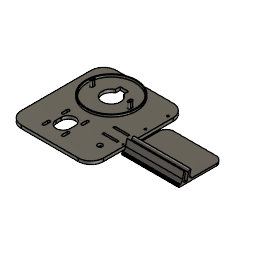
Nasty_Mounting (Autodesk Fusion 360 design; units mm, degrees)
Autodesk Fusion 360 part; units mm, degrees
sketch "bovenkant" plane through (0, 0, 0) normal (0, 0, 1) x (1, 0, 0)
  circle A0 centre (-96.358, 36.4115) radius 1.25
  circle A1 centre (-48.858, 36.4115) radius 1.25
  circle A2 centre (-96.358, -11.0885) radius 1.25
  circle A3 centre (-48.858, -11.0885) radius 1.25
  circle A4 centre (-72.6345, 12.688) radius 14.5
  line L0 (-66.1493, 33.1295) -> (-79.0952, 33.1295)
  line L1 (-79.0952, 33.1295) -> (-79.0952, 25.6691)
  line L2 (-66.1493, 25.6569) -> (-66.1493, 33.1295)
  line L3 (-72.6345, 12.688) -> (-74.3845, 12.688)
  line L4 (-72.6345, 12.688) -> (-70.8845, 12.688)
  line L5 (-104.9345, 14.288) -> (-104.9345, 11.088)
  arc A5 (-104.9345, 11.088) -> (-100.1345, 11.088) centre (-102.5345, 11.088) ccw
  line L6 (-100.1345, 11.088) -> (-100.1345, 14.288)
  arc A6 (-100.1345, 14.288) -> (-104.9345, 14.288) centre (-102.5345, 14.288) ccw
  arc A7 (-104.6845, 11.088) -> (-100.3845, 11.088) centre (-102.5345, 11.088) ccw
  line L7 (-100.3845, 11.088) -> (-100.3845, 14.2881)
  arc A8 (-100.3845, 14.2881) -> (-104.6845, 14.288) centre (-102.5345, 14.288) ccw
  line L8 (-104.6845, 14.288) -> (-104.6845, 11.088)
  arc A9 (-71.0345, -19.612) -> (-71.0345, -14.812) centre (-71.0345, -17.212) ccw
  line L9 (-71.0345, -14.812) -> (-74.2345, -14.812)
  arc A10 (-74.2345, -15.062) -> (-74.2345, -19.362) centre (-74.2345, -17.212) ccw
  arc A11 (-71.0345, -19.362) -> (-71.0345, -15.062) centre (-71.0345, -17.212) ccw
  line L10 (-74.2345, -19.362) -> (-71.0345, -19.362)
  line L11 (-74.2345, -19.612) -> (-71.0345, -19.612)
  arc A12 (-74.2345, -14.812) -> (-74.2345, -19.612) centre (-74.2345, -17.212) ccw
  line L12 (-71.0345, -15.062) -> (-74.2345, -15.062)
  arc A13 (-40.3345, 14.288) -> (-45.1345, 14.288) centre (-42.7345, 14.288) ccw
  line L13 (-45.1345, 14.288) -> (-45.1345, 11.088)
  arc A14 (-44.8845, 11.088) -> (-40.5845, 11.088) centre (-42.7345, 11.088) ccw
  arc A15 (-40.5845, 14.2881) -> (-44.8845, 14.288) centre (-42.7345, 14.288) ccw
  line L14 (-40.5845, 11.088) -> (-40.5845, 14.2881)
  line L15 (-40.3345, 11.088) -> (-40.3345, 14.288)
  arc A16 (-45.1345, 11.088) -> (-40.3345, 11.088) centre (-42.7345, 11.088) ccw
  line L16 (-44.8845, 14.288) -> (-44.8845, 11.088)
  arc A17 (-74.2345, 44.988) -> (-74.2345, 40.188) centre (-74.2345, 42.588) ccw
  line L17 (-74.2345, 40.188) -> (-71.0345, 40.188)
  arc A18 (-71.0345, 40.438) -> (-71.0345, 44.738) centre (-71.0345, 42.588) ccw
  arc A19 (-74.2345, 44.738) -> (-74.2345, 40.438) centre (-74.2345, 42.588) ccw
  line L18 (-71.0345, 44.738) -> (-74.2345, 44.738)
  line L19 (-71.0345, 44.988) -> (-74.2345, 44.988)
  arc A20 (-71.0345, 40.188) -> (-71.0345, 44.988) centre (-71.0345, 42.588) ccw
  line L20 (-74.2345, 40.438) -> (-71.0345, 40.438)
  circle A21 centre (-72.6345, 12.688) radius 37.5
  circle A22 centre (-72.6345, 12.688) radius 39.75
  circle A23 centre (-102.5345, 12.688) radius 1.6
  circle A24 centre (-42.7345, 12.688) radius 1.6
  point P0 (-72.6345, 12.688)
  point P1 (-72.6345, 12.688)
  dimension "d4" = 2.5
  dimension "d7" = 47.5
  dimension "d8" = -47.5
  dimension "d9" = 29
  dimension "d12" = 7.4725
  dimension "d19" = -0.25
  dimension "d21" = 360
  dimension "d22" = 27.5
  dimension "d23" = 75
  dimension "d24" = 79.5
  dimension "d41" = 360
  dimension "d44" = 3.2
  constraint horizontal L0
  constraint perpendicular L0 L1
  constraint parallel L1 L2
  constraint coincident P1 P0
  constraint coincident A4 L1.end
  constraint coincident A4 L2.start
  constraint horizontal L3
  constraint coincident P0 A4.centre
  constraint horizontal L4
  constraint tangent L5 A5
  constraint tangent A5 L6
  constraint parallel L5 L6
  constraint tangent L6 A6
  constraint tangent L5 A6
  constraint coincident A5.centre A23
  constraint coincident A6.centre A23
  measures "d4" diameter of A0
  measures "d9" diameter of A4
  measures "d12" distance of L0.start L2.start
  measures "d22" distance of P1 L6
  measures "d23" diameter of A21
  measures "d24" diameter of A22
  measures "d44" diameter of A23
extrude "Extrude1" add sketch "bovenkant" against normal blind 3 contours A0 | A1 | A2 | A3 | A4 | A4 L0 L1 L2 | L5 A5 L6 A6 | A7 L7 A8 L8 | A9 L9 L11 A12 | A10 A11 L10 L12 | A13 L13 L15 A16 | A14 A15 L14 L16 | A17 L17 L19 A20 | A18 A19 L18 L20 | A21 | A22 | A23 | A24 makes body 1
extrude "Extrude3" add sketch "bovenkant" along normal blind 9 separate body contours A7 L7 A8 L8 | A14 A15 L14 L16 | A23 | A24 makes body 2 at (-42.1522, 9.0184, 3) makes body 3 at (-102.1611, 16.4054, 6)
ref_plane "WorkPlane1" through (-96.358, 36.4115, 3) normal (0, 0, 1) x (1, 0, 0)
sketch "rand" plane through (0, 0, 3) normal (0, 0, 1) x (1, 0, 0)
  circle A0 centre (-72.6345, 12.688) radius 39.75
  circle A1 centre (-72.6345, 12.688) radius 38.25
  dimension "d32" = -1.5
extrude "Extrude4" add sketch "rand" against normal up to surface (3 mm away) bodies 1
chamfer "Chamfer1" distance 0.5 distance2 3 1 edges at (-108.296, -1.1438, 0) measured on face at (-75.4716, 23.995, 0) on bodies 1
extrude "Extrude5" cut sketch "bovenkant" against normal up to surface (3 mm away) contours A4 | A4 L0 L1 L2 bodies 1
combine "Combine1" operation add target body 3 tool bodies 1 2
extrude "Extrude6" cut sketch "bovenkant" along normal blind 14 and the other way blind 2 contours A23 | A24 bodies 3
sketch "Onderkant" plane through (0, 0, -3) normal (0, 0, -1) x (1, 0, 0)
  arc A0 (-66.1493, -25.6569) -> (-79.0952, -25.6691) centre (-72.6345, -12.688) ccw
  line L0 (-66.1493, -25.6569) -> (-66.1493, -33.1295)
  line L1 (-66.1493, -33.1295) -> (-79.0952, -33.1295)
  line L2 (-79.0952, -33.1295) -> (-79.0952, -25.6691)
  circle A1 centre (-72.6345, -12.688) radius 39.75
  circle A2 centre (-42.7345, -12.688) radius 1.6
  circle A3 centre (-102.5345, -12.688) radius 1.6
  line L3 (-45.6345, -14.3624) -> (-42.7345, -16.0367)
  line L4 (-42.7345, -16.0367) -> (-39.8345, -14.3624)
  line L5 (-39.8345, -14.3624) -> (-39.8345, -11.0137)
  line L6 (-39.8345, -11.0137) -> (-42.7345, -9.3394)
  line L7 (-42.7345, -9.3394) -> (-45.6345, -11.0137)
  line L8 (-45.6345, -11.0137) -> (-45.6345, -14.3624)
  line L9 (-105.4345, -14.3624) -> (-102.5345, -16.0367)
  line L10 (-102.5345, -16.0367) -> (-99.6345, -14.3624)
  line L11 (-99.6345, -14.3624) -> (-99.6345, -11.0137)
  line L12 (-99.6345, -11.0137) -> (-102.5345, -9.3394)
  line L13 (-102.5345, -9.3394) -> (-105.4345, -11.0137)
  line L14 (-105.4345, -11.0137) -> (-105.4345, -14.3624)
  point P0 (-102.5345, -12.688)
  point P1 (-42.7345, -12.688)
  point P2 (-42.7345, -12.688)
  point P3 (-102.5345, -12.688)
  dimension "d45" = 2.9
  dimension "d46" = 2.9
  constraint coincident P2 P1
  constraint coincident P3 P0
  measures "d45" distance of P2 L8
  measures "d46" distance of P3 L14
sketch "maten_hardware" plane through (0, 0, 0) normal (0, 0, 1) x (1, 0, 0)
  circle A0 centre (-72.6345, 12.688) radius 39.75
  circle A1 centre (-72.6345, 12.688) radius 39.75
  line L0 (-83.9345, -55.312) -> (-83.9345, -63.312)
  arc A2 (-83.9345, -63.312) -> (-61.4345, -63.312) centre (-72.6845, -63.312) ccw
  line L1 (-61.4345, -63.312) -> (-61.4345, -55.312)
  arc A3 (-61.4345, -55.312) -> (-83.9345, -55.312) centre (-72.6845, -55.312) ccw
  line L2 (-72.6845, -55.312) -> (-72.6845, -63.312) construction
  line L3 (-57.4289, -44.062) -> (-57.4289, -40.062)
  line L4 (-57.4289, -44.062) -> (-57.4289, -48.062)
  line L5 (-59.3289, -40.062) -> (-59.3289, -48.062)
  arc A4 (-59.3289, -48.062) -> (-55.5289, -48.062) centre (-57.4289, -48.062) ccw
  line L6 (-55.5289, -48.062) -> (-55.5289, -40.062)
  arc A5 (-55.5289, -40.062) -> (-59.3289, -40.062) centre (-57.4289, -40.062) ccw
  line L7 (-57.4289, -40.062) -> (-57.4289, -48.062) construction
  line L8 (-50.6309, -20.4164) -> (-50.6309, -84.1336)
  line L9 (-50.6309, -84.1336) -> (-94.6381, -84.1336)
  line L10 (-94.6381, -84.1336) -> (-94.6381, -20.4164)
  line L11 (-87.9289, -44.062) -> (-87.9289, -48.062)
  line L12 (-87.9289, -40.062) -> (-87.9289, -48.062) construction
  line L13 (-87.9289, -44.062) -> (-87.9289, -40.062)
  line L14 (-86.0289, -48.062) -> (-86.0289, -40.062)
  arc A6 (-86.0289, -40.062) -> (-89.8289, -40.062) centre (-87.9289, -40.062) ccw
  line L15 (-89.8289, -40.062) -> (-89.8289, -48.062)
  arc A7 (-89.8289, -48.062) -> (-86.0289, -48.062) centre (-87.9289, -48.062) ccw
  line L16 (-57.4289, -74.562) -> (-57.4289, -78.562)
  line L17 (-57.4289, -70.562) -> (-57.4289, -78.562) construction
  line L18 (-57.4289, -74.562) -> (-57.4289, -70.562)
  line L19 (-55.5289, -78.562) -> (-55.5289, -70.562)
  arc A8 (-55.5289, -70.562) -> (-59.3289, -70.562) centre (-57.4289, -70.562) ccw
  line L20 (-59.3289, -70.562) -> (-59.3289, -78.562)
  arc A9 (-59.3289, -78.562) -> (-55.5289, -78.562) centre (-57.4289, -78.562) ccw
  line L21 (-87.9289, -74.562) -> (-87.9289, -78.562)
  line L22 (-87.9289, -70.562) -> (-87.9289, -78.562) construction
  line L23 (-87.9289, -74.562) -> (-87.9289, -70.562)
  line L24 (-86.0289, -78.562) -> (-86.0289, -70.562)
  arc A10 (-86.0289, -70.562) -> (-89.8289, -70.562) centre (-87.9289, -70.562) ccw
  line L25 (-89.8289, -70.562) -> (-89.8289, -78.562)
  arc A11 (-89.8289, -78.562) -> (-86.0289, -78.562) centre (-87.9289, -78.562) ccw
  line L26 (4.0655, -25.2683) -> (-32.3045, -25.2683)
  line L27 (-32.3045, -25.2683) -> (-32.3045, -45.5883)
  line L28 (-32.3045, -45.5883) -> (4.0655, -45.5883)
  line L29 (4.0655, -45.5883) -> (4.0655, -25.2683)
  line L30 (2.0955, -27.2683) -> (2.0955, -43.5883)
  line L31 (-29.9045, -28.7883) -> (-29.9045, -42.0683)
  circle A12 centre (2.0955, -27.2683) radius 1.15
  circle A13 centre (-29.9045, -28.7883) radius 1.15
  circle A14 centre (-29.9045, -42.0683) radius 1.15
  circle A15 centre (2.0955, -43.5883) radius 1.15
  circle A16 centre (-1.1507, 30.6175) radius 1.6
  circle A17 centre (-36.6507, 30.6175) radius 1.6
  circle A18 centre (-1.1507, -4.8825) radius 1.6
  circle A19 centre (-36.6507, -4.8825) radius 1.6
  line L32 (2.5993, 34.3675) -> (-40.4007, 34.3675)
  line L33 (-40.4007, 34.3675) -> (-40.4007, -8.6325)
  line L34 (-40.4007, -8.6325) -> (2.5993, -8.6325)
  line L35 (2.5993, -8.6325) -> (2.5993, 34.3675)
  line L36 (-8.6345, -56.7369) -> (-21.1345, -56.7369)
  line L37 (-21.1345, -56.7369) -> (-21.1345, -69.2369)
  line L38 (-21.1345, -69.2369) -> (-8.6345, -69.2369)
  line L39 (-8.6345, -69.2369) -> (-8.6345, -56.7369)
  line L40 (-8.6345, -56.7369) -> (-21.1345, -69.2369) construction
  line L41 (-21.1345, -56.7369) -> (-8.6345, -69.2369) construction
  circle A20 centre (-14.8845, -62.9869) radius 3.75
  line L42 (-96.0345, 6.5117) -> (-123.6345, 6.5117)
  line L43 (-123.6345, 6.5117) -> (-123.6345, -57.4883)
  line L44 (-123.6345, -57.4883) -> (-96.0345, -57.4883)
  line L45 (-96.0345, -57.4883) -> (-96.0345, 6.5117)
  line L46 (-29.1045, -25.3683) -> (-5.6045, -25.3683)
  line L47 (-5.6045, -25.3683) -> (-5.6045, -28.3683)
  line L48 (-5.6045, -28.3683) -> (-29.1045, -28.3683)
  line L49 (-29.1045, -28.3683) -> (-29.1045, -25.3683)
  line L50 (-31.2285, -35.4283) -> (-20.6732, -35.4283)
  line L51 (-5.6045, -42.4883) -> (-29.1045, -42.4883)
  line L52 (-29.1045, -42.4883) -> (-29.1045, -45.4883)
  line L53 (-29.1045, -45.4883) -> (-5.6045, -45.4883)
  line L54 (-5.6045, -45.4883) -> (-5.6045, -42.4883)
  line L55 (5.3655, -77.4883) -> (5.3655, 32.5117)
  line L56 (-14.6345, 52.5117) -> (-104.6345, 52.5117)
  line L57 (-124.6345, 32.5117) -> (-124.6345, -77.4883)
  line L58 (-104.6345, -97.4883) -> (-14.6345, -97.4883)
  arc A21 (-104.6345, 52.5117) -> (-124.6345, 32.5117) centre (-104.6345, 32.5117) ccw
  arc A22 (5.3655, 32.5117) -> (-14.6345, 52.5117) centre (-14.6345, 32.5117) ccw
  arc A23 (-124.6345, -77.4883) -> (-104.6345, -97.4883) centre (-104.6345, -77.4883) ccw
  arc A24 (-14.6345, -97.4883) -> (5.3655, -77.4883) centre (-14.6345, -77.4883) ccw
  point P0 (-72.6845, -59.312)
  point P1 (-14.8845, -62.9869)
  point P2 (5.3655, -97.4883)
  point P3 (-124.6345, -97.4883)
  dimension "d53" = 22.5
  dimension "d57" = 4
  dimension "d58" = 4
  dimension "d63" = 3.8
  dimension "d80" = -30.5
  dimension "d81" = -30.5
  dimension "d82" = 36.37
  dimension "d83" = 20.32
  dimension "d88" = 16.32
  dimension "d89" = 2
  dimension "d90" = 1.97
  dimension "d91" = 13.28
  dimension "d92" = 3.52
  dimension "d93" = 2.4
  dimension "d94" = 2.3
  dimension "d95" = 2.3
  dimension "d97" = 2.3
  dimension "d98" = 2.3
  dimension "d102" = 3.2
  dimension "d105" = -35.5
  dimension "d106" = -35.5
  dimension "d107" = 43
  dimension "d108" = 43
  dimension "d109" = 3.75
  dimension "d110" = 3.75
  dimension "d111" = 12.5
  dimension "d112" = 12.5
  dimension "d113" = 7.5
  dimension "d114" = 27.6
  dimension "d115" = 64
  dimension "d118" = 23.5
  dimension "d119" = 3
  dimension "d120" = 0.1
  dimension "d121" = 3.2
  dimension "d122" = 10.16
  dimension "d123" = 130
  dimension "d124" = 20
  dimension "d139" = 150
  dimension "d140" = 1.3
  dimension "d147" = 2.7662
  dimension "d148" = 1
  dimension "d149" = 44.0072
  dimension "d150" = 52
  dimension "d151" = 14
  dimension "d152" = 52
  dimension "d153" = 40
  constraint tangent L0 A2
  constraint tangent A2 L1
  constraint parallel L0 L1
  constraint tangent L1 A3
  constraint tangent L0 A3
  constraint midpoint L2 P0
  constraint tangent L5 A4
  constraint tangent A4 L6
  constraint parallel L5 L6
  constraint tangent L6 A5
  constraint tangent L5 A5
  constraint coincident L4.end A4.centre
  constraint parallel L4 L7
  constraint coincident L3.end A5.centre
  constraint perpendicular L8 L9
  constraint parallel L8 L10
  constraint coincident A1 L8.start
  constraint horizontal L26
  constraint vertical L27
  constraint horizontal L28
  constraint vertical L29
  constraint perpendicular L26 L30
  constraint perpendicular L26 L31
  constraint coincident L30.start A12.centre
  constraint coincident L31.start A13.centre
  constraint coincident L31.end A14.centre
  constraint coincident L30.end A15.centre
  constraint horizontal L32
  constraint vertical L33
  constraint horizontal L34
  constraint vertical L35
  constraint horizontal L36
  constraint perpendicular L36 L37
  constraint parallel L36 L38
  constraint parallel L37 L39
  constraint coincident L40 P1
  constraint coincident L41 P1
  constraint coincident P1 A20.centre
  constraint horizontal L42
  constraint vertical L43
  constraint horizontal L44
  constraint vertical L45
  constraint horizontal L46
  constraint vertical L47
  constraint horizontal L48
  constraint vertical L49
  constraint horizontal L50
  constraint symmetric L46.start L50 L52.end
  constraint symmetric L46.end L50 L53.end
  constraint symmetric L47.end L50 L51.start
  constraint symmetric L48.end L50 L51.end
  constraint perpendicular L55 L56
  constraint parallel L55 L57
  constraint parallel L56 L58
  constraint perpendicular L32 L55
  constraint tangent L56 A21
  constraint tangent L57 A21
  constraint tangent L55 A22
  constraint tangent L56 A22
  constraint equal A21 A22
  constraint coincident P3 L57
  constraint coincident P3 L58
  constraint tangent L57 A23
  constraint tangent L58 A23
  constraint equal A21 A23
  constraint coincident P2 L55
  constraint coincident P2 L58
  constraint tangent L55 A24
  constraint tangent L58 A24
  constraint equal A21 A24
  constraint coincident A0 L10.end
  measures "d53" diameter of A2
  measures "d57" distance of L3.start L3.end
  measures "d58" distance of L3.start L4.end
  measures "d63" diameter of A4
  measures "d82" distance of L26.start L26.end
  measures "d83" distance of L26.start L28.end
  measures "d88" distance of L30.start L30.end
  measures "d89" distance of L26 L30.start
  measures "d90" distance of L29 L30
  measures "d91" distance of L31.start L31.end
  measures "d92" distance of L26 L31.start
  measures "d93" distance of L27 L31
  measures "d94" diameter of A12
  measures "d95" diameter of A13
  measures "d97" diameter of A14
  measures "d98" diameter of A15
  measures "d102" diameter of A16
  measures "d107" distance of L32.start L32.end
  measures "d108" distance of L32.start L34.end
  measures "d109" distance of A16.centre L35
  measures "d110" distance of A16.centre L32
  measures "d111" distance of L37.end L38.end
  measures "d112" distance of L36.end L37.end
  measures "d113" diameter of A20
  measures "d114" distance of L42.start L42.end
  measures "d115" distance of L42.start L44.end
  measures "d118" distance of L46.start L46.end
  measures "d119" distance of L46.start L48.end
  measures "d120" distance of L26 L46
  measures "d121" distance of L27 L49
  measures "d122" distance of L26 L50
  measures "d123" distance of P2 P3
  measures "d124" radius of A21
  measures "d139" distance of L56 L58
  measures "d140" distance of L29 L55
  measures "d147" distance of L35 L55
  measures "d148" distance of L43 L57
  measures "d149" distance of L8 L10
  measures "d150" distance of A0.centre L57
  measures "d151" distance of L39 L55
  measures "d152" distance of L53 L58
  measures "d153" distance of L44 L58
extrude "Extrude8" add sketch "maten_hardware" against normal blind 5 contours A0 A1 L8 L9 L10 | A0 A1 L42 L43 L44 L45 | A0 A1 A17 A19 L32 L34 L35 | A0 A1 A19 | A0 A1 A17 | L26 L27 L28 L29 | A13 L48 L49 | A14 L51 L52 | L36 L37 L38 L39 | L55 L56 L57 L58 A21 A22 A23 A24 picked at (-36.348, -5.0254) picked at (-36.4402, 30.7083) picked at (-30.3145, -29.0044) picked at (-30.3145, -41.8522) bodies 3
extrude "Extrude12" add 1 faces at (-71.6362, 39.5286, -3) along direction (0, 0, -1) up to surface (2 mm away) on bodies 3 bodies 3
ref_plane "WorkPlane2" through (-59.6345, -22.4883, -5) normal (0, 0, -1) x (-1, 0, 0)
sketch "Sketch6" plane through (0, 0, -5) normal (0, 0, -1) x (-1, 0, 0)
  line L0 (123.6345, -57.4883) -> (96.0345, -57.4883)
  line L1 (123.6345, 6.5117) -> (123.6345, -57.4883)
  line L2 (96.0345, -57.4883) -> (96.0345, 6.5117)
  line L3 (96.0345, 6.5117) -> (123.6345, 6.5117)
  line L4 (8.6345, -56.7369) -> (21.1345, -56.7369)
  line L5 (21.1345, -56.7369) -> (21.1345, -69.2369)
  line L6 (21.1345, -69.2369) -> (8.6345, -69.2369)
  line L7 (8.6345, -69.2369) -> (8.6345, -56.7369)
  line L8 (40.4007, -8.6325) -> (-2.5993, -8.6325)
  line L9 (40.4007, 34.3675) -> (40.4007, -8.6325)
  line L10 (-2.5993, 34.3675) -> (40.4007, 34.3675)
  line L11 (-2.5993, -8.6325) -> (-2.5993, 34.3675)
extrude "Extrude10" cut sketch "Sketch6" against normal blind 3.5 bodies 3
sketch "Sketch7" plane through (0, 0, 0) normal (1, 0, 0) x (0, 1, 0)
  line L0 (-91.4917, 4.5771) -> (-93.4917, 4.5771)
  line L1 (-93.9917, 4.0771) -> (-93.9917, -66.1853)
  line L2 (-93.9917, -66.1853) -> (-90.9917, -66.1853)
  line L3 (-90.9917, 2.1282) -> (-90.9917, 4.0771)
  arc A0 (-90.9917, 2.1282) -> (-90.5352, 1.6301) centre (-90.4917, 2.1282) ccw
  arc A1 (-90.9917, 4.0771) -> (-91.4917, 4.5771) centre (-91.4917, 4.0771) ccw
  arc A2 (-93.4917, 4.5771) -> (-93.9917, 4.0771) centre (-93.4917, 4.0771) ccw
  line L4 (-90.9917, -0.4229) -> (-75.3696, -3.8798)
  line L5 (-77.8019, -14.8716) -> (-93.4104, -11.4098)
  line L6 (-93.4104, -11.4098) -> (-90.9917, -0.4229)
  line L7 (-77.152, -11.9349) -> (-91.7977, -8.6941)
  line L8 (-91.7977, -8.6941) -> (-90.6634, -3.5681)
  line L9 (-90.6634, -3.5681) -> (-76.0177, -6.8089)
  line L10 (-75.3696, -3.8798) -> (-76.0177, -6.8089)
  line L11 (-77.152, -11.9349) -> (-77.8019, -14.8716)
  line L12 (-90.8603, 1.7904) -> (-90.9917, -66.1853)
  point P0 (-90.9917, 4.5771)
  point P1 (-93.9917, 4.5771)
  dimension "d131" = 3
  dimension "d134" = 0.5
  dimension "d160" = 16
  dimension "d161" = 11.25
  dimension "d162" = 15
  dimension "d163" = 5.25
  dimension "d164" = 3
  dimension "d165" = 3
  dimension "d166" = 5
  constraint horizontal L0
  constraint vertical L1
  constraint horizontal L2
  constraint tangent L3 A0
  constraint coincident P0 L0
  constraint coincident P0 L3
  constraint tangent L0 A1
  constraint tangent L3 A1
  constraint equal A0 A1
  constraint coincident P1 L0
  constraint coincident P1 L1
  constraint tangent L0 A2
  constraint tangent L1 A2
  constraint equal A0 A2
  constraint parallel L7 L9
  constraint coincident L7.start L10
  constraint collinear L10 L11
  constraint midpoint A0 L12.start
  measures "d131" distance of P0 P1
  measures "d134" radius of A0
  measures "d160" distance of L4.start L4.end
  measures "d161" distance of L4.start L5.end
  measures "d162" distance of L9.end L8.end
  measures "d163" distance of L7 L9
  measures "d164" distance of L4 L9
  measures "d165" distance of L1 L4.start
  measures "d166" distance of L0 L4.start
extrude "Extrude11" add sketch "Sketch7" along normal blind 90 separate body contours L0 L1 L2 L3 A0 A1 A2 L4 L5 L6 L12 | L4 L5 L6 L7 L8 L12 | L4 L8 L9 L10 L12 | L5 L7 L11 L12 makes body 4
fillet "Fillet2" radius 10 tangency weight 0.62362 2 edges at (0, -92.4917, -66.1853) (90, -92.4917, -66.1853) on bodies 4
extrude "Extrude13" add 1 faces at (-14.7911, -57.5738, -1.5) along direction (0, 0, -1) blind 2 on bodies 3 bodies 3
fillet "Fillet3" radius 4 2 edges at (45, -77.152, -11.9349) (45, -76.0177, -6.8089) on bodies 4
fillet "Fillet4" radius 4 1 edges at (45, -90.8869, -11.9695) on bodies 4
fillet "Fillet5" radius 9.5 1 edges at (45, -90.8646, -0.451) on bodies 4
move_body "Move1" bodies 4 to x (1, 0, 0) y (0, 0, 1) z (0, -1, 0) at (12.5014, -51.5144, 91.0064)
equation "d88 = d83 - 4 mm"
equation "d89 = ( d83 - d88 ) / 2"
equation "d91 = d83 - ( ( 2 * 3.52 ) * 1 mm )"
equation "d92 = ( d83 - d91 ) / 2"
equation "d94 = Gat_esp32"
equation "d95 = Gat_esp32"
equation "Gat_esp32 = 2.3 mm"
equation "d97 = Gat_esp32"
equation "d98 = Gat_esp32"
equation "gat_stepper = 3.2 mm"
equation "d102 = gat_stepper"
equation "d109 = ( d107 - 35.5 mm ) / 2"
equation "d110 = ( d108 - 35.5 mm ) / 2"
equation "d114 = stroombreed"
equation "d115 = stroomhoog"
equation "stroomhoog = 64 mm"
equation "stroombreed = 27.6 mm"
equation "d122 = d83 / 2"
equation "d161 = 5.25 mm + 6 mm"
equation "d165 = d131"
named bodies: "Mounting Plate", "Stand"
